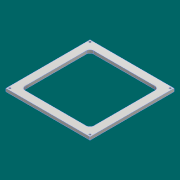
# Autodesk Inventor part: spacer
Saved by Autodesk Inventor 2016 (Build 200138000, 138)
## iProperties
Created: 2016-06-17
Part Number: spacer
Material: Aluminum 6061
Document SubType Name: Modeling
Designer: sawaiz
Density: 2.7 g/cm^3
Appearance: Aluminum - Flat
Author: sawaiz
Autodesk Inventor part; units mm, degrees
ref_plane "YZ Plane" through (0, 0, 0) normal (1, 0, 0) x (0, 1, 0)
ref_plane "XZ Plane" through (0, 0, 0) normal (0, 1, 0) x (-1, 0, 0)
ref_plane "XY Plane" through (0, 0, 0) normal (0, 0, 1) x (1, 0, 0)
sketch "Sketch1" plane through (0, 0, 0) normal (0, 0, 1) x (1, 0, 0)
  line L0 (-63.5, -63.5) -> (63.5, -63.5)
  line L1 (63.5, -63.5) -> (63.5, 63.5)
  line L2 (63.5, 63.5) -> (-63.5, 63.5)
  line L3 (-63.5, 63.5) -> (-63.5, -63.5)
  line L4 (-63.5, -63.5) -> (63.5, 63.5) construction
  line L5 (63.5, -63.5) -> (-63.5, 63.5) construction
  line L6 (-69.85, -69.85) -> (69.85, -69.85)
  line L7 (69.85, -69.85) -> (69.85, 69.85)
  line L8 (69.85, 69.85) -> (-69.85, 69.85)
  line L9 (-69.85, 69.85) -> (-69.85, -69.85)
  line L10 (-57.15, -57.15) -> (57.15, -57.15)
  line L11 (57.15, -57.15) -> (57.15, 57.15)
  line L12 (57.15, 57.15) -> (-57.15, 57.15)
  line L13 (-57.15, 57.15) -> (-57.15, -57.15)
  point P0 (0, 0)
  dimension "d0" = 127
  dimension "d1" = 127
  dimension "d2" = 6.35
  dimension "d3" = 6.35
  constraints: 28 end point, 6 parallel, 3 perpendicular, 2 midpoint, 1 horizontal, 6 other
  measures "d0" distance of L2.end L1.end
  measures "d1" distance of L1.end L0.end
  measures "d2" distance between parallel lines of L3 L9
  measures "d3" distance between parallel lines of L3 L13
extrude "Extrusion1" add sketch "Sketch1" along normal blind 5.08 contours L3 L2 L1 L0 | L9 L8 L7 L6
sketch "Sketch2" plane through (0, 0, 5.08) normal (0, 0, 1) x (1, 0, 0)
  line L0 (-57.15, -57.15) -> (-57.15, 57.15) projected
  line L1 (-57.15, 57.15) -> (57.15, 57.15) projected
  line L2 (57.15, 57.15) -> (57.15, -57.15) projected
  line L3 (57.15, -57.15) -> (-57.15, -57.15) projected
  line L4 (-69.85, -69.85) -> (69.85, -69.85) projected
  line L5 (69.85, -69.85) -> (69.85, 69.85) projected
  line L6 (69.85, 69.85) -> (-69.85, 69.85) projected
  line L7 (-69.85, 69.85) -> (-69.85, -69.85) projected
  point P0 (0, 0)
  point P1 (-66.675, 66.675)
  dimension "d6" = 3.175
  dimension "d7" = 3.175
  measures "d6" distance from line of L7 point (-66.675, 66.675)
  measures "d7" distance from line of L6 point (-66.675, 66.675)
hole "Hole1" at (-66.675, 66.675, 5.08) direction (0, 0, -1) diameter 3.264 end through all clearance for "Flat Head Machine Screw (82)" size "#4" standard "Ansi Unified Screw Threads"
mirror "Mirror1" about plane through (0, 0, 0) normal (0, 1, 0) of "Hole1"
mirror "Mirror2" about plane through (0, 0, 0) normal (1, 0, 0) of "Hole1", "Mirror1"
fillet "Fillet1" radius 6.35 4 edges at (-57.15, 57.15, 2.54) (57.15, 57.15, 2.54) (-57.15, -57.15, 2.54) (57.15, -57.15, 2.54)
body "Solid1"
